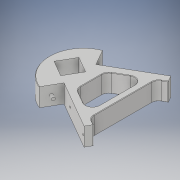
# Autodesk Inventor part: Profil_Winkel
Saved by Autodesk Inventor 2019 (Build 230136000, 136)
## iProperties
Created: 2018-08-17
Part Number: Profil_Winkel
Material: Generic
Document SubType Name: Modeling
Designer: Julia
Density: 1 g/cm^3
Appearance: Default
Author: Julia
Autodesk Inventor part; units mm, degrees
ref_plane "YZ Plane" through (0, 0, 0) normal (1, 0, 0) x (0, 1, 0)
ref_plane "XZ Plane" through (0, 0, 0) normal (0, 1, 0) x (-1, 0, 0)
ref_plane "XY Plane" through (0, 0, 0) normal (0, 0, 1) x (1, 0, 0)
sketch "Sketch1" plane through (0, 0, 0) normal (0, 1, 0) x (-1, 0, 0)
  line L0 (-126.3701, 48.161) -> (-51.2671, 4.8003) construction
  line L1 (-51.2671, 4.8003) -> (-126.3701, -38.5605) construction
  line L2 (-126.3701, -38.5605) -> (-126.3701, 48.161) construction
  line L3 (110.9585, 0) -> (-59.5814, 0) construction
  line L4 (83.2089, 69.641) -> (63.2089, 35)
  line L5 (63.2089, 35) -> (-40.7142, 95)
  line L6 (-40.7142, 95) -> (-48.2142, 82.0096)
  line L7 (-48.2142, 82.0096) -> (-30.8937, 72.0096)
  line L8 (-17.9033, 64.5096) -> (38.3884, 32.0096)
  line L9 (83.2089, -69.641) -> (63.2089, -35)
  line L10 (63.2089, -35) -> (-40.7142, -95)
  line L11 (-40.7142, -95) -> (-48.2142, -82.0096)
  line L12 (-48.2142, -82.0096) -> (-30.8937, -72.0096)
  line L13 (-17.9033, -64.5096) -> (38.3884, -32.0096)
  arc A0 (83.2089, -69.641) -> (83.2089, 69.641) centre (55.3678, 0) ccw
  line L14 (-30.8937, 72.0096) -> (-30.8937, -72.0096)
  line L15 (-17.9033, 64.5096) -> (-17.9033, -64.5096)
  line L16 (38.3884, 32.0096) -> (38.3884, -32.0096)
  dimension "d3" = 40
  dimension "d4" = 120
  dimension "d5" = 15
  dimension "d7" = 20
  dimension "d19" = 70
  dimension "d20" = 75
  dimension "d21" = 15
  dimension "d22" = 65
  constraints: 34 end point, 7 symmetric about line, 5 vertical, 4 perpendicular, 2 equal length, 2 horizontal, 2 point on circle, 1 centre point, 1 collinear, 1 parallel, 1 point on line, 3 other
  measures "d3" distance of L4.start L4.end
  measures "d4" distance of L4.end L5.end
  measures "d5" distance of L5.end L6.end
  measures "d7" distance of L6.end L7.end
  measures "d19" distance of L9.end L4.end
  measures "d20" radius of A0
  measures "d21" distance of L8.start L7.end
  measures "d22" distance of L8.start L8.end
extrude "Extrusion1" add sketch "Sketch1" along normal blind 40
sketch "Sketch2" plane through (-63.2089, 0, 35) normal (0.8660254, 0, 0.5) x (0.5, 0, -0.8660254)
  circle A0 centre (-20, 20) radius 3.4
  line L0 (-40, 40) -> (0, 40) projected
  line L1 (-40, 0) -> (-40, 40) projected
  point P0 (61.9153, 0)
  point P1 (-20, 40)
  point P2 (-40, 20)
  dimension "d10" = 6.8
  constraints: 2 midpoint, 1 centre point, 1 horizontal alignment, 1 vertical alignment
  measures "d10" diameter of A0
extrude "Extrusion2" add sketch "Sketch2" along normal blind 10
sketch "Sketch3" plane through (-83.2089, 0, -69.641) normal (0.8660254, 0, -0.5) x (-0.5, 0, -0.8660254)
  circle A0 centre (-20, 20) radius 3.4
  line L0 (-40, 40) -> (0, 40) projected
  line L1 (0, 0) -> (0, 40) projected
  point P0 (-101.9153, 0)
  point P1 (-20, 40)
  point P2 (0, 20)
  dimension "d13" = 6.8
  constraints: 2 midpoint, 1 centre point, 1 horizontal alignment, 1 vertical alignment
  measures "d13" diameter of A0
extrude "Extrusion3" add sketch "Sketch3" along normal blind 10
sketch "Sketch4" plane through (0, 40, 0) normal (0, 1, 0) x (1, 0, 0)
  line L0 (-115.1704, -5) -> (-80.5294, -25)
  line L1 (-80.5294, -25) -> (-60.5294, 9.641)
  line L2 (-60.5294, 9.641) -> (-95.1704, 29.641)
  line L3 (-95.1704, 29.641) -> (-115.1704, -5)
  line L4 (-38.3884, -32.0096) -> (-38.3884, 32.0096) projected
  line L5 (-63.2089, -35) -> (40.7142, -95) projected
  line L6 (-83.2089, -69.641) -> (-63.2089, -35) projected
  point P0 (0, 0)
  point P1 (-105.1704, 12.3205)
  dimension "d16" = 40
  dimension "d17" = 40
  dimension "d49" = 20
  constraints: 8 end point, 3 parallel, 2 collinear, 1 midpoint, 1 perpendicular
  measures "d16" distance of L2.end L0.start
  measures "d17" distance of L1.end L2.end
  measures "d49" distance of L0.end L5.start
extrude "Extrusion4" cut sketch "Sketch4" against normal blind 40
fillet "Fillet1" radius 15 2 edges at (-38.3884, 20, -32.0096) (-38.3884, 20, 32.0096)
fillet "Fillet2" radius 15 2 edges at (17.9033, 20, 64.5096) (17.9033, 20, -64.5096)
fillet "Fillet3" radius 15 2 edges at (30.8937, 20, 72.0096) (30.8937, 20, -72.0096)
sketch "Sketch5" plane through (48.2142, 0, 82.0096) normal (0.5, 0, -0.8660254) x (-0.8660254, 0, -0.5)
  point P0 (82.7595, 0)
  point P1 (5.815, 19.918)
hole "Hole1" at (43.1783, 19.918, 79.1021) direction (-0.5, 0, 0.8660254) diameter 4 end through all counterbore diameter 5 counterbore depth 2
sketch "Sketch6" plane through (-30.8884, 0, 36.3397) normal (0.5, 0, -0.8660254) x (-0.8660254, 0, -0.5)
  point P0 (-8.5802, 0)
  point P1 (-7.7378, 18.9937)
hole "Hole2" at (-24.1872, 18.9937, 40.2087) direction (-0.5, 0, 0.8660254) diameter 4 end through all counterbore diameter 5 counterbore depth 2
fillet "Fillet8" radius 1 28 edges at (-36.3788, 0, 30.8494) (-17.7426, 0, 43.9295) (10.4033, 0, 51.5192) (17.9033, 0, 0) (10.4033, 0, -51.5192) (-17.7426, 0, -43.9295) (-36.3788, 0, -30.8494) (-38.3884, 0, 0) (32.9033, 0, -70.8494) (43.3039, 0, -79.1747) (32.9033, 0, 70.8494) (43.3039, 0, 79.1747) (30.8937, 0, 0) (-36.3788, 40, -30.8494) (-17.7426, 40, -43.9295) (10.4033, 40, -51.5192) (17.9033, 40, 0) (10.4033, 40, 51.5192) (-17.7426, 40, 43.9295) (-36.3788, 40, 30.8494) (-38.3884, 40, 0) (32.9033, 40, -70.8494) (43.3039, 40, -79.1747) (32.9033, 40, 70.8494) (43.3039, 40, 79.1747) (30.8937, 40, 0) (48.2142, 20, 82.0096) (48.2142, 20, -82.0096)
fillet "Fillet9" radius 1 2 edges at (-130.3678, 0, 0) (-130.3678, 40, 0)
body "Solid1"
